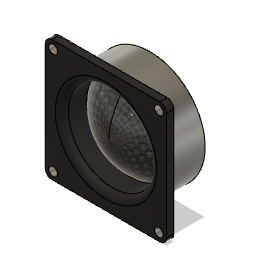
Main v23 (Autodesk Fusion 360 archive; units mm, degrees)
design "Monacor DT-28N"
Autodesk Fusion 360 part; units mm, degrees
sketch "Skizze1" plane through (0, 0, 0) normal (1, 0, 0) x (0, 0, -1)
  line L0 (16.7, 25) -> (16.7, 0)
  line L1 (16.7, 0) -> (0, 0)
  line L2 (16.7, 25) -> (-3.3, 25)
  line L3 (-3.3, 25) -> (-3.3, 23)
  line L4 (-0.3, 20) -> (8, 20)
  spline S0 degree 2 poles (8, 20) (-1.5, 11) (-2, 0) knots 0 0 0 2.280457 2.280457 2.280457
  arc A0 (-3.3, 23) -> (-0.3, 20) centre (-0.3, 23) ccw
  line L5 (0, 0) -> (-2, 0)
  dimension "d5" = 3.3
  dimension "d6" = 20
  dimension "d8" = 25
  dimension "d24" = 3
  dimension "d25" = 8
  dimension "d26" = 2
  dimension "d27" = 5
  dimension "d28" = 9
  dimension "d29" = 1.5
  constraint coincident L1.end L5.start
  constraint perpendicular L0 L1
  constraint perpendicular L0 L2
  constraint horizontal L2
  constraint perpendicular L2 L3
  constraint perpendicular L3 L4
  constraint tangent L3 A0
  constraint tangent L4 A0
  constraint parallel L1 L5
  measures "d5" horizontal distance of L1.end L2.end
  measures "d6" distance of L0.start L2.end
  measures "d8" vertical distance of L1.end L2.end
  measures "d24" radius of A0
  measures "d25" horizontal distance of L1.end L4.end
  measures "d26" distance of L1.end S0.end
  measures "d27" distance of L2 L4.end
revolve "Drehen1" add sketch "Skizze1" angle 360 about axis through (0, 0, 1.75) along (0, 0, 1)
sketch "Skizze2" plane through (0, 0, 3.3) normal (0, 0, 1) x (1, 0, 0)
  circle A0 centre (0, 0) radius 20
  circle A1 centre (0, 0) radius 25
  line L0 (24.5, -27.5) -> (-24.5, -27.5)
  line L1 (-27.5, -24.5) -> (-27.5, 24.5)
  line L2 (-24.5, 27.5) -> (24.5, 27.5)
  line L3 (27.5, 24.5) -> (27.5, -24.5)
  line L4 (27.5, -27.5) -> (-27.5, 27.5) construction
  line L5 (-27.5, -27.5) -> (27.5, 27.5) construction
  line L6 (24, -24) -> (-24, -24) construction
  line L7 (-24, -24) -> (-24, 24) construction
  line L8 (-24, 24) -> (24, 24) construction
  line L9 (24, 24) -> (24, -24) construction
  line L10 (24, -24) -> (-24, 24) construction
  line L11 (-24, -24) -> (24, 24) construction
  circle A2 centre (24, 24) radius 2
  circle A3 centre (-24, 24) radius 2
  circle A4 centre (-24, -24) radius 2
  circle A5 centre (24, -24) radius 2
  arc A6 (27.5, 24.5) -> (24.5, 27.5) centre (24.5, 24.5) ccw
  arc A7 (-24.5, 27.5) -> (-27.5, 24.5) centre (-24.5, 24.5) ccw
  arc A8 (-27.5, -24.5) -> (-24.5, -27.5) centre (-24.5, -24.5) ccw
  arc A9 (24.5, -27.5) -> (27.5, -24.5) centre (24.5, -24.5) ccw
  circle A10 centre (0, 0) radius 23
  circle A11 centre (0, 0) radius 25
  dimension "d11" = 55
  dimension "d12" = 55
  dimension "d13" = 48
  dimension "d14" = 48
  dimension "d15" = 4
  dimension "d17" = 360
  dimension "d18" = 3
  dimension "d19" = 3
  dimension "d20" = 3
  dimension "d21" = 3
  constraint perpendicular L0 L1
  constraint parallel L0 L2
  constraint parallel L1 L3
  constraint horizontal L0
  constraint coincident L4 A0.centre
  constraint coincident L5 A0.centre
  constraint coincident A0.centre A1.centre
  constraint perpendicular L6 L7
  constraint parallel L6 L8
  constraint parallel L7 L9
  constraint horizontal L6
  constraint coincident L10 A0.centre
  constraint coincident L11 A0.centre
  constraint coincident L8.end L9.start
  constraint coincident L5.end L3
  constraint coincident L5.end L2
  constraint tangent L3 A6
  constraint tangent L2 A6
  constraint coincident L4.end L2
  constraint coincident L4.end L1
  constraint tangent L2 A7
  constraint tangent L1 A7
  constraint coincident L5.start L1
  constraint coincident L5.start L0
  constraint tangent L1 A8
  constraint tangent L0 A8
  constraint coincident L4.start L0
  constraint coincident L4.start L3
  constraint tangent L0 A9
  constraint tangent L3 A9
  measures "d11" distance of L4.end L5.end
  measures "d12" distance of L5.start L4.end
  measures "d13" distance of L7.end L8.end
  measures "d14" distance of L6.end L7.end
  measures "d15" diameter of A2
  measures "d18" radius of A6
  measures "d19" radius of A7
  measures "d20" radius of A8
  measures "d21" radius of A9
extrude "Extrusion1" add sketch "Skizze2" against normal blind 3.3 contours L0 L1 L2 L3 A6 A7 A8 A9
named bodies: "Main"

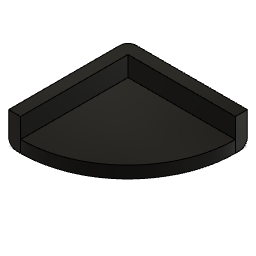
design "Corner"
Autodesk Fusion 360 part; units mm, degrees
sketch "Skizze1" plane through (0, 0, 0) normal (0, 1, 0) x (1, 0, 0)
  line L0 (0, 0) -> (0, -30)
  line L1 (0, 0) -> (30, 0)
  line L2 (0, -30) -> (3, -30)
  line L3 (3, -30) -> (3, -3)
  line L4 (3, -3) -> (30, -3)
  line L5 (30, -3) -> (30, 0)
  arc A0 (3, -30) -> (30, -3) centre (3, -3) ccw
  line L6 (3, -3) -> (3, -30) construction
  line L7 (3, -3) -> (30, -3) construction
  point P0 (3, -3)
  dimension "d1" = 30
  dimension "d2" = 30
  dimension "d4" = 27
  dimension "d5" = 27
  dimension "d6" = 90
  constraint coincident L0.start L1.start
  constraint vertical L0
  constraint horizontal L1
  constraint perpendicular L0 L2
  constraint perpendicular L2 L3
  constraint horizontal L4
  constraint vertical L5
  constraint coincident P0 L3.end
  measures "d1" distance of L0.start L0.end
  measures "d2" distance of L0.start L1.end
  measures "d4" distance of L2.end P0
  measures "d5" distance of P0 L4.end
  measures "d6" angle of L6 L7
extrude "Extrusion1" add sketch "Skizze1" against normal blind 3
extrude "Extrusion2" add sketch "Skizze1" along normal blind 5 contours L0 L1 L2 L3 L4 L5
fillet "Abrundung1" radius 2 3 edges at (0, 1, 0) (0, -3, 15) (15, -3, 0)
named bodies: "Main"

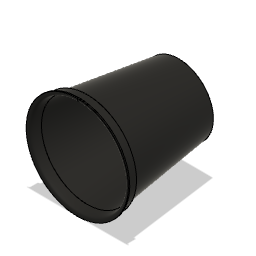
design "Monacor BR-100HP"
Autodesk Fusion 360 part; units mm, degrees
sketch "Skizze1" plane through (0, 0, 0) normal (1, 0, 0) x (0, 0, -1)
  line L0 (-1.8, 71.5) -> (0, 71.5)
  line L1 (0, 71.5) -> (0, 69)
  line L2 (0, 69) -> (12, 69)
  line L3 (12, 69) -> (12, 66)
  line L4 (12, 66) -> (140, 48.5186)
  line L5 (140, 48.5186) -> (140, 46.5)
  line L6 (140, 46.5) -> (12, 63.9814)
  spline S0 degree 2 poles (12, 63.9814) (-1.3, 65.7979) (-1.8, 71.5) knots 0 0 0 1.729263 1.729263 1.729263 weights 1 2.333333 1
  dimension "d1" = 71.5
  dimension "d2" = 2.5
  dimension "d3" = 3
  dimension "d4" = 2
  dimension "d5" = 140
  dimension "d6" = 1.8
  dimension "d7" = 12
  dimension "d8" = 46.5
  dimension "d9" = 1.3
  constraint perpendicular L0 L1
  constraint perpendicular L1 L2
  constraint perpendicular L2 L3
  constraint perpendicular L2 L5
  constraint parallel L4 L6
  constraint coincident origin L1
  constraint vertical L1
  constraint coincident L3 L6.end
  measures "d1" distance of origin L0.end
  measures "d2" distance of L0.end L1.end
  measures "d3" distance of L2.end L3.end
  measures "d4" distance of L4 L6
  measures "d5" horizontal distance of L0.end L4.end
  measures "d6" distance of L0.start L0.end
  measures "d7" distance of L1.end L2.end
  measures "d8" vertical distance of origin L5.end
revolve "Drehen1" add sketch "Skizze1" angle 360 about axis through (0, 0, 1.75) along (0, 0, 1)
equation "d1 = ( 143 / 2 ) * 1 mm"
equation "d2 = ( ( 143 - 138 ) / 2 ) * 1 mm"
equation "d8 = ( 93 / 2 ) * 1 mm"
named bodies: "Main"

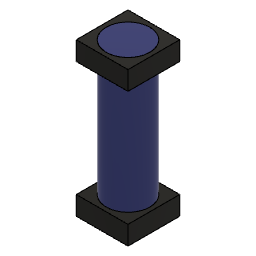
design "Cell"
Autodesk Fusion 360 part; units mm, degrees
sketch "Skizze1" plane through (0, 0, 0) normal (0, 1, 0) x (1, 0, 0)
  line L0 (11, -11) -> (-11, -11)
  line L1 (-11, -11) -> (-11, 11)
  line L2 (-11, 11) -> (11, 11)
  line L3 (11, 11) -> (11, -11)
  line L4 (11, -11) -> (-11, 11) construction
  line L5 (-11, -11) -> (11, 11) construction
  circle A0 centre (0, 0) radius 9.25
  dimension "d1" = 22
  dimension "d2" = 22
  dimension "d3" = 18.5
  constraint perpendicular L0 L1
  constraint parallel L0 L2
  constraint parallel L1 L3
  constraint horizontal L0
  constraint coincident L4 A0.centre
  constraint coincident L5 A0.centre
  constraint coincident A0.centre origin
  measures "d1" distance of L0.end L1.end
  measures "d2" distance of L1.end L2.end
  measures "d3" diameter of A0
extrude "Extrusion1" add sketch "Skizze1" along normal blind 65 contours A0 makes body 1
extrude "Extrusion2" add sketch "Skizze1" along normal blind 8 separate body makes body 2
copy_body "Körper kopieren/einfügen1" bodies 2 makes body 3
move_body "Verschieben2" bodies 3 to x (1, 0, 0) y (0, 1, 0) z (0, 0, 1) at (0, 57, 0)

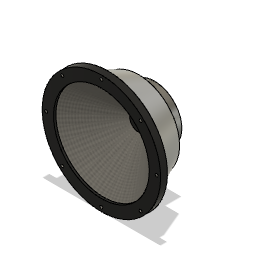
design "Beyma 10BR60V2"
Autodesk Fusion 360 part; units mm, degrees
sketch "Skizze1" plane through (0, 0, 0) normal (1, 0, 0) x (0, 0, -1)
  line L0 (67, 20) -> (67, 0)
  line L1 (67, 0) -> (102, 0)
  line L2 (102, 0) -> (102, 60)
  line L3 (102, 60) -> (67, 60)
  line L4 (-15, 130.25) -> (-15, 105.25)
  line L5 (-15, 105.25) -> (-10, 105.25)
  line L6 (-10, 105.25) -> (67, 20)
  line L7 (0, 130.25) -> (0, 114)
  line L8 (0, 130.25) -> (-15, 130.25)
  line L9 (67, 60) -> (67, 90)
  line L10 (0, 114) -> (10, 114)
  line L11 (10, 114) -> (67, 90)
  dimension "d1" = 114
  dimension "d2" = 20
  dimension "d4" = 15
  dimension "d5" = 5
  dimension "d7" = 16.25
  dimension "d8" = 102
  dimension "d9" = 35
  dimension "d10" = 60
  dimension "d11" = 30
  dimension "d12" = 25
  dimension "d22" = 10
  constraint perpendicular L0 L1
  constraint perpendicular L1 L2
  constraint perpendicular L2 L3
  constraint perpendicular L4 L5
  constraint coincident origin L1
  constraint perpendicular L4 L8
  constraint vertical L7
  constraint horizontal L8
  constraint coincident origin L7
  constraint horizontal L3
  constraint perpendicular L3 L9
  constraint collinear L0 L9
  constraint perpendicular L7 L10
  measures "d1" vertical distance of origin L7.end
  measures "d2" vertical distance of origin L0.start
  measures "d4" distance of L7.start L4.start
  measures "d5" distance of L4.end L5.end
  measures "d7" distance of L7.start L7.end
  measures "d8" distance of origin L1.end
  measures "d9" distance of L2.end L3.end
  measures "d10" distance of L1.end L2.end
  measures "d11" distance of L3.end L9.end
  measures "d12" distance of L4.start L4.end
  measures "d22" distance of L7.end L10.end
revolve "Drehen1" add sketch "Skizze1" angle 360 about axis through (0, 0, 1.75) along (0, 0, 1)
sketch "Skizze2" plane through (0, 0, 15) normal (0, 0, 1) x (1, 0, 0)
  circle A0 centre (0, 0) radius 105.25
  circle A1 centre (0, 0) radius 130.25
  circle A2 centre (0, 0) radius 121.75 construction
  circle A3 centre (0, 121.75) radius 3.1
  line L0 (0, 0) -> (0, 140) construction
  circle A4 centre (-86.0903, 86.0903) radius 3.1
  circle A5 centre (-121.75, 0) radius 3.1
  circle A6 centre (-86.0903, -86.0903) radius 3.1
  circle A7 centre (0, -121.75) radius 3.1
  circle A8 centre (86.0903, -86.0903) radius 3.1
  circle A9 centre (121.75, 0) radius 3.1
  circle A10 centre (86.0903, 86.0903) radius 3.1
  dimension "d14" = 243.5
  dimension "d16" = 6.2
  dimension "d17" = 140
  dimension "d19" = 360
  constraint coincident A0.centre A1.centre
  constraint coincident A2 A3.centre
  constraint vertical L0
  constraint coincident A3.centre L0
  measures "d14" diameter of A2
  measures "d16" diameter of A3
  measures "d17" distance of A0.centre L0.end
extrude "Extrusion1" cut sketch "Skizze2" against normal blind 20 contours A3 | A4 | A5 | A6 | A7 | A8 | A9 | A10
equation "d1 = ( 228 / 2 ) * 1 mm"
named bodies: "Main"

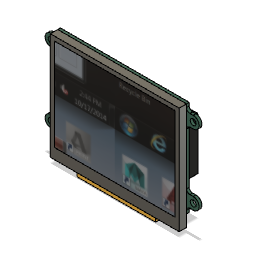
design "NHD-3.5-320240FT-CSXN-T"
Autodesk Fusion 360 part; units mm, degrees
sketch "Skizze1" plane through (0, 0, 0) normal (0, 0, 1) x (1, 0, 0)
  line L0 (0, 0) -> (76.9, 0)
  line L1 (76.9, 0) -> (76.9, 63.9)
  line L2 (76.9, 63.9) -> (0, 63.9)
  line L3 (0, 63.9) -> (0, 0)
  line L4 (0, 31.95) -> (76.9, 31.95) construction
  line L5 (0, 35.45) -> (76.9, 35.45) construction
  circle A0 centre (-4, 14.45) radius 1.75
  line L6 (38.45, 0) -> (38.45, 63.9) construction
  line L7 (74.36, 6.31) -> (2.54, 6.31)
  line L8 (2.54, 6.31) -> (2.54, 61.36)
  line L9 (2.54, 61.36) -> (74.36, 61.36)
  line L10 (74.36, 61.36) -> (74.36, 6.31)
  line L11 (74.36, 6.31) -> (2.54, 61.36) construction
  line L12 (2.54, 6.31) -> (74.36, 61.36) construction
  line L13 (15, 0) -> (15, -3)
  line L14 (15, -3) -> (61.9, -3)
  line L15 (61.9, -3) -> (61.9, 0)
  line L16 (76.9, 7) -> (0, 7)
  line L17 (15, 7) -> (15, 0)
  line L18 (61.9, 0) -> (61.9, 7)
  line L19 (-2, 18) -> (-4, 18)
  arc A1 (-4, 18) -> (-7.55, 14.45) centre (-4, 14.45) ccw
  line L20 (-4, 14.45) -> (-4, 18) construction
  line L21 (-4, 14.45) -> (-7.55, 14.45) construction
  arc A2 (-7.55, 14.45) -> (-4, 10.9) centre (-4, 14.45) ccw
  line L22 (-4, 14.45) -> (-7.55, 14.45) construction
  line L23 (-4, 14.45) -> (-4, 10.9) construction
  line L24 (-4, 10.9) -> (-2, 10.9)
  arc A3 (-2, 18) -> (0, 20) centre (-2, 20) ccw
  arc A4 (0, 8.9) -> (-2, 10.9) centre (-2, 8.9) ccw
  arc A5 (-4, 60) -> (-7.55, 56.45) centre (-4, 56.45) ccw
  line L25 (-4, 56.45) -> (-7.55, 56.45) construction
  arc A6 (-2, 60) -> (0, 62) centre (-2, 62) ccw
  line L26 (-4, 56.45) -> (-4, 52.9) construction
  arc A7 (0, 50.9) -> (-2, 52.9) centre (-2, 50.9) ccw
  circle A8 centre (-4, 56.45) radius 1.75
  line L27 (-4, 56.45) -> (-4, 60) construction
  line L28 (-4, 56.45) -> (-7.55, 56.45) construction
  line L29 (-2, 52.9) -> (-4, 52.9)
  line L30 (-4, 60) -> (-2, 60)
  arc A9 (-7.55, 56.45) -> (-4, 52.9) centre (-4, 56.45) ccw
  line L31 (80.9, 14.45) -> (84.45, 14.45) construction
  line L32 (78.9, 18) -> (80.9, 18)
  circle A10 centre (80.9, 14.45) radius 1.75
  arc A11 (84.45, 14.45) -> (80.9, 18) centre (80.9, 14.45) ccw
  line L33 (80.9, 14.45) -> (84.45, 14.45) construction
  arc A12 (78.9, 10.9) -> (76.9, 8.9) centre (78.9, 8.9) ccw
  line L34 (80.9, 14.45) -> (80.9, 10.9) construction
  line L35 (80.9, 14.45) -> (80.9, 18) construction
  arc A13 (76.9, 20) -> (78.9, 18) centre (78.9, 20) ccw
  line L36 (80.9, 10.9) -> (78.9, 10.9)
  arc A14 (80.9, 10.9) -> (84.45, 14.45) centre (80.9, 14.45) ccw
  line L37 (80.9, 56.45) -> (84.45, 56.45) construction
  arc A15 (78.9, 52.9) -> (76.9, 50.9) centre (78.9, 50.9) ccw
  line L38 (80.9, 56.45) -> (84.45, 56.45) construction
  arc A16 (84.45, 56.45) -> (80.9, 60) centre (80.9, 56.45) ccw
  arc A17 (80.9, 52.9) -> (84.45, 56.45) centre (80.9, 56.45) ccw
  line L39 (80.9, 56.45) -> (80.9, 52.9) construction
  line L40 (80.9, 60) -> (78.9, 60)
  arc A18 (76.9, 62) -> (78.9, 60) centre (78.9, 62) ccw
  line L41 (78.9, 52.9) -> (80.9, 52.9)
  line L42 (80.9, 56.45) -> (80.9, 60) construction
  circle A19 centre (80.9, 56.45) radius 1.75
  point P0 (-2, 62)
  point P1 (76.9, 31.95)
  point P2 (76.9, 35.45)
  point P3 (38.45, 33.835)
  point P4 (78.9, 62)
  dimension "d1" = 76.9
  dimension "d2" = 63.9
  dimension "d18" = 28.45
  dimension "d23" = 3.5
  dimension "d24" = 21
  dimension "d26" = 42.45
  dimension "d29" = 71.82
  dimension "d30" = 55.05
  dimension "d31" = 2.54
  dimension "d34" = 3
  dimension "d35" = 15
  dimension "d36" = 7
  dimension "d39" = 46
  dimension "d40" = 15.45
  constraint horizontal L0
  constraint horizontal L2
  constraint vertical L3
  constraint coincident L0.start L3.end
  constraint midpoint L3 L4.start
  constraint midpoint L1 P1
  constraint coincident L3 L5.start
  constraint coincident L1 P2
  constraint perpendicular L1 L5
  constraint midpoint L0 L6.start
  constraint midpoint L2 L6.end
  constraint symmetric L4.start L6 P1
  constraint symmetric L5.start L6 P2
  constraint perpendicular L7 L8
  constraint parallel L7 L9
  constraint parallel L8 L10
  constraint horizontal L7
  constraint coincident L11 P3
  constraint coincident L12 P3
  constraint coincident L6 P3
  constraint coincident L0 L13.start
  constraint perpendicular L0 L13
  constraint perpendicular L13 L14
  constraint coincident L0 L15.end
  constraint perpendicular L0 L15
  constraint symmetric L6 L13 L15
  constraint coincident L1 L16.start
  constraint coincident L3 L16.end
  constraint perpendicular L3 L16
  constraint coincident L16 L18.end
  constraint perpendicular L16 L18
  constraint coincident L16 L17.start
  constraint collinear L13 L17
  constraint coincident A0.centre A1.centre
  constraint vertical L20
  constraint horizontal L21
  constraint vertical L23
  constraint tangent L19 A1
  constraint tangent A2 L24
  constraint coincident L3 A3.end
  constraint tangent L19 A3
  constraint tangent L3 A3
  constraint coincident L3 A4.start
  constraint tangent L24 A4
  constraint tangent L3 A4
  constraint equal L19 L24
  constraint symmetric L5 L19.start A7.end
  constraint symmetric L5 A0 A8
  constraint symmetric L5 L24.end A6.start
  constraint symmetric L5 L19.end L26.end
  constraint symmetric L5 A1.end A5.end
  constraint symmetric L5 A1 A9
  constraint symmetric L5 A2.end A5.start
  constraint symmetric L5 A2 A5
  constraint symmetric L5 A3.end A7.start
  constraint symmetric L5 A3 A7
  constraint symmetric L5 A4.start A6.end
  constraint symmetric L5 A4 A6
  constraint symmetric L19.start L6 L32.start
  constraint symmetric A0 L6 A10
  constraint symmetric L6 L24.end A12.start
  constraint symmetric L6 P0 P4
  constraint symmetric L6 L19.end L32.end
  constraint symmetric L6 A1.end L31.end
  constraint symmetric L6 A1 A11
  constraint symmetric L6 A2.end L34.end
  constraint symmetric L6 A2 A14
  constraint symmetric L6 A3.end A13.start
  constraint symmetric L6 A3 A13
  constraint symmetric L6 A4.start A12.end
  constraint symmetric L6 A4 A12
  constraint symmetric L6 A5.end L37.end
  constraint symmetric L6 L26.end A17.start
  constraint symmetric L6 A6.start L40.end
  constraint symmetric L6 A7.start A15.end
  constraint symmetric L6 A7.end A15.start
  constraint symmetric L6 A6.end A18.start
  constraint symmetric L6 A5.start A16.end
  constraint symmetric L6 A5 A16
  constraint symmetric L6 A6 A18
  constraint symmetric L6 A7 A15
  constraint symmetric L6 A8 A19
  constraint symmetric L6 A9 A17
  measures "d1" distance of L0.start L0.end
  measures "d2" distance of L0.start L2.end
  measures "d18" distance of L2 L5
  measures "d23" diameter of A0
  measures "d24" distance of L5 A0.centre
  measures "d26" distance of A0.centre L6
  measures "d29" distance of L8.end L9.end
  measures "d30" distance of L7.end L8.end
  measures "d31" distance of L2 L8.end
  measures "d34" distance of L13.start L13.end
  measures "d35" distance of L0.start L13.start
  measures "d36" distance of L0.start L16.end
  measures "d39" distance of L6 A1.end
  measures "d40" distance of L5 A3.end
extrude "Extrusion3" add sketch "Skizze1" along normal blind 3.5 contours L0 L13 L14 L15 makes body 1
extrude "Extrusion4" add sketch "Skizze1" against normal blind 1.6 contours L0 L7 L17 L18 | L0 L13 L14 L15 | L7 L16 L17 L18 bodies 1
extrude "Extrusion5" add sketch "Skizze1" against normal blind 1.6 separate body contours L1 L2 L3 L8 L9 L10 L16 | L3 L19 A1 A2 L24 A3 A4 | L8 L9 L10 L16 | L3 A5 A6 A7 L29 L30 A9 | L1 L32 A11 A12 A13 L36 A14 | L1 A15 A16 A17 L40 A18 L41 makes body 2
extrude "Extrusion6" add sketch "Skizze1" along normal blind 4.4 separate body contours L0 L3 L7 L8 L16 L17 | L0 L7 L17 L18 | L1 L2 L3 L8 L9 L10 L16 | L0 L1 L7 L10 L16 L18 makes body 3
extrude "Extrusion7" add sketch "Skizze1" along normal blind 4.4 separate body contours L7 L16 L17 L18 | L7 L8 L16 L17 | L8 L9 L10 L16 | L7 L10 L16 L18 makes body 4
sketch "Skizze2" plane through (0, 0, -1.6) normal (0, 0, -1) x (-1, 0, 0)
  circle A0 centre (4, 14.45) radius 1.75
  circle A1 centre (-80.9, 56.45) radius 1.75
  circle A2 centre (4, 56.45) radius 1.75
  circle A3 centre (-80.9, 14.45) radius 1.75
  line L0 (-76.9, 50.9) -> (-76.9, 20)
  arc A4 (-78.9, 18) -> (-76.9, 20) centre (-78.9, 20) ccw
  line L1 (-78.9, 18) -> (-80.9, 18)
  arc A5 (-80.9, 18) -> (-80.9, 10.9) centre (-80.9, 14.45) ccw
  line L2 (-80.9, 10.9) -> (-78.9, 10.9)
  arc A6 (-76.9, 8.9) -> (-78.9, 10.9) centre (-78.9, 8.9) ccw
  line L3 (-76.9, 8.9) -> (-76.9, 7)
  line L4 (-76.9, 7) -> (0, 7)
  line L5 (0, 7) -> (0, 8.9)
  arc A7 (2, 10.9) -> (0, 8.9) centre (2, 8.9) ccw
  line L6 (2, 10.9) -> (4, 10.9)
  arc A8 (4, 10.9) -> (4, 18) centre (4, 14.45) ccw
  line L7 (4, 18) -> (2, 18)
  arc A9 (0, 20) -> (2, 18) centre (2, 20) ccw
  line L8 (0, 20) -> (0, 50.9)
  arc A10 (2, 52.9) -> (0, 50.9) centre (2, 50.9) ccw
  line L9 (2, 52.9) -> (4, 52.9)
  arc A11 (4, 52.9) -> (4, 60) centre (4, 56.45) ccw
  line L10 (4, 60) -> (2, 60)
  arc A12 (0, 62) -> (2, 60) centre (2, 62) ccw
  line L11 (0, 62) -> (0, 63.9)
  line L12 (0, 63.9) -> (-76.9, 63.9)
  line L13 (-76.9, 63.9) -> (-76.9, 62)
  arc A13 (-78.9, 60) -> (-76.9, 62) centre (-78.9, 62) ccw
  line L14 (-78.9, 60) -> (-80.9, 60)
  arc A14 (-80.9, 60) -> (-80.9, 52.9) centre (-80.9, 56.45) ccw
  line L15 (-80.9, 52.9) -> (-78.9, 52.9)
  arc A15 (-76.9, 50.9) -> (-78.9, 52.9) centre (-78.9, 50.9) ccw
  line L16 (-72.4, 50.9) -> (-64.4, 50.9)
  line L17 (-64.4, 50.9) -> (-64.4, 20)
  line L18 (-64.4, 20) -> (-72.4, 20)
  line L19 (-72.4, 20) -> (-72.4, 50.9)
  line L20 (-76.9, 35.45) -> (0, 35.45) construction
  line L21 (-61.9, 50.9) -> (-15, 50.9)
  line L22 (-15, 50.9) -> (-15, -3)
  line L23 (-15, -3) -> (-61.9, -3)
  line L24 (-61.9, -3) -> (-61.9, 50.9)
  line L25 (0, 47.95) -> (-7, 47.95)
  line L26 (-7, 47.95) -> (-7, 22.95)
  line L27 (-7, 22.95) -> (0, 22.95)
  line L28 (0, 22.95) -> (0, 47.95)
  point P0 (-72.4, 35.45)
  point P1 (-61.9, -3)
  point P2 (-15, -3)
  dimension "d55" = 8
  dimension "d56" = 30.9
  dimension "d57" = 4.5
  dimension "d58" = 7
  dimension "d59" = 25
  constraint horizontal L16
  constraint vertical L17
  constraint horizontal L18
  constraint vertical L19
  constraint midpoint L0 L20.start
  constraint midpoint L8 L20.end
  constraint midpoint L19 P0
  constraint coincident L20 P0
  constraint horizontal L21
  constraint vertical L22
  constraint horizontal L23
  constraint vertical L24
  constraint coincident P1 L23.end
  constraint coincident P2 L22.end
  constraint collinear L16 L21
  constraint horizontal L25
  constraint vertical L26
  constraint horizontal L27
  constraint vertical L28
  constraint coincident L8 L25.start
  constraint midpoint L20.end L28
  measures "d55" distance of L16.start L16.end
  measures "d56" distance of L16.start L18.end
  measures "d57" distance of L0 L18.end
  measures "d58" distance of L26.end L27.end
  measures "d59" distance of L25.end L26.end
extrude "Extrusion8" add sketch "Skizze2" along normal blind 9.8 separate body contours L16 L17 L18 L19 makes body 5
extrude "Extrusion9" add sketch "Skizze2" along normal blind 2 separate body contours L8 L25 L26 L27 L28 makes body 6
extrude "Extrusion10" add sketch "Skizze2" along normal blind 2 separate body contours L4 L21 L22 L24 | L4 L22 L23 L24 makes body 7
combine "Kombinieren1" operation add target body 1 tool bodies 7
equation "d26 = ( 84.9 / 2 ) * 1 mm"
equation "d36 = 63.9 mm - 56.9 mm"
equation "d39 = ( 92 / 2 ) * 1 mm"
equation "d40 = ( 30.9 / 2 ) * 1 mm"
equation "d60 = 11.4 mm - 1.6 mm"
named bodies: "FFCPlaceholder", "PCB", "MetalFrame", "LCD", "IDC Connector", "FFC Connector"

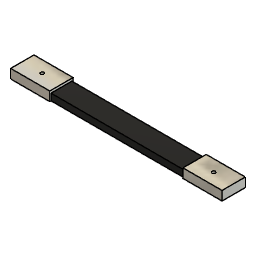
design "Handle"
Autodesk Fusion 360 part; units mm, degrees
sketch "Skizze1" plane through (0, 0, 0) normal (0, 1, 0) x (1, 0, 0)
  line L0 (80, -12.5) -> (-80, -12.5)
  line L1 (-80, -12.5) -> (-80, 12.5)
  line L2 (-80, 12.5) -> (80, 12.5)
  line L3 (80, 12.5) -> (80, -12.5)
  line L4 (80, -12.5) -> (-80, 12.5) construction
  line L5 (-80, -12.5) -> (80, 12.5) construction
  line L6 (80, 14) -> (127, 14)
  line L7 (127, 14) -> (127, -14)
  line L8 (127, -14) -> (80, -14)
  line L9 (80, -14) -> (80, 14)
  line L10 (0, 12.5) -> (0, -12.5) construction
  line L11 (80, 0) -> (127, 0) construction
  circle A0 centre (103, 0) radius 2
  line L12 (-80, 0) -> (-127, 0) construction
  line L13 (-127, -14) -> (-80, -14)
  circle A1 centre (-103, 0) radius 2
  line L14 (-127, 14) -> (-127, -14)
  line L15 (-80, 14) -> (-127, 14)
  line L16 (-80, -14) -> (-80, 14)
  dimension "d1" = 160
  dimension "d2" = 25
  dimension "d3" = 28
  dimension "d4" = 47
  dimension "d5" = 4
  dimension "d6" = 103
  constraint perpendicular L0 L1
  constraint parallel L0 L2
  constraint parallel L1 L3
  constraint horizontal L0
  constraint coincident L4 origin
  constraint coincident L5 origin
  constraint horizontal L6
  constraint vertical L7
  constraint horizontal L8
  constraint vertical L9
  constraint midpoint L3 L9
  constraint midpoint L2 L10.start
  constraint midpoint L0 L10.end
  constraint midpoint L9 L11.start
  constraint midpoint L7 L11.end
  constraint coincident L11 A0.centre
  constraint symmetric L6.start L10 L15.start
  constraint symmetric L6.end L10 L14.start
  constraint symmetric L7.end L10 L13.start
  constraint symmetric L8.end L10 L13.end
  constraint symmetric L10 L11.start L12.start
  constraint symmetric L10 L11.end L12.end
  constraint symmetric L10 A0 A1
  measures "d1" distance of L1.end L2.end
  measures "d2" distance of L0.end L1.end
  measures "d3" distance of L6.start L8.end
  measures "d4" distance of L6.start L6.end
  measures "d5" diameter of A0
  measures "d6" distance of origin A0.centre
extrude "Extrusion1" add sketch "Skizze1" along normal blind 11 contours L3 L6 L7 L8 L9 | L1 L13 L14 L15 L16 makes body 1 at (-119.6667, 0, 0) makes body 2 at (119.6667, 0, 0)
extrude "Extrusion2" add sketch "Skizze1" along normal blind 8 separate body contours L0 L1 L2 L3 L9 L16 makes body 3
equation "d4 = ( ( 254 - 160 ) / 2 ) * 1 mm"
named bodies: "End1", "End2", "Center"

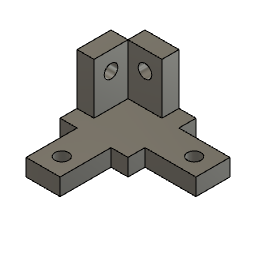
design "2020 Corner Piece"
Autodesk Fusion 360 part; units mm, degrees
sketch "Skizze1" plane through (0, 0, 0) normal (0, 1, 0) x (1, 0, 0)
  line L0 (0, 0) -> (20, 0)
  line L1 (0, 0) -> (0, -20)
  line L2 (0, -20) -> (5, -20)
  line L3 (5, -20) -> (5, -35)
  line L4 (5, -35) -> (15, -35)
  line L5 (15, -35) -> (15, -20)
  line L6 (15, -20) -> (20, -20)
  line L7 (20, -20) -> (20, -15)
  line L8 (20, -15) -> (35, -15)
  line L9 (35, -15) -> (35, -5)
  line L10 (35, -5) -> (20, -5)
  line L11 (20, -5) -> (20, 0)
  line L12 (35, -10) -> (0, -10) construction
  line L13 (10, 0) -> (10, -35) construction
  circle A0 centre (29.5, -10) radius 2
  circle A1 centre (10, -29.5) radius 2
  dimension "d3" = 20
  dimension "d4" = 20
  dimension "d5" = 5
  dimension "d6" = 15
  dimension "d7" = 10
  dimension "d8" = 15
  dimension "d9" = 10
  dimension "d10" = 5
  dimension "d11" = 4
  dimension "d12" = 5.5
  dimension "d13" = 4
  dimension "d14" = 5.5
  constraint horizontal L0
  constraint coincident L0.start L1.start
  constraint perpendicular L0 L1
  constraint perpendicular L1 L2
  constraint perpendicular L2 L3
  constraint perpendicular L3 L4
  constraint perpendicular L4 L5
  constraint perpendicular L5 L6
  constraint perpendicular L6 L7
  constraint perpendicular L7 L8
  constraint perpendicular L8 L9
  constraint perpendicular L9 L10
  constraint collinear L2 L6
  constraint collinear L7 L11
  constraint midpoint L9 L12.start
  constraint midpoint L1 L12.end
  constraint midpoint L0 L13.start
  constraint midpoint L4 L13.end
  constraint coincident L12 A0.centre
  constraint coincident L13 A1.centre
  measures "d3" distance of L0.start L0.end
  measures "d4" distance of L0.start L1.end
  measures "d5" distance of L1.end L2.end
  measures "d6" distance of L2.end L3.end
  measures "d7" distance of L3.end L4.end
  measures "d8" distance of L7.end L8.end
  measures "d9" distance of L8.end L9.end
  measures "d10" distance of L0.end L10.end
  measures "d11" diameter of A0
  measures "d12" distance of L9 A0.centre
  measures "d13" diameter of A1
  measures "d14" distance of L4 A1.centre
extrude "Extrusion1" add sketch "Skizze1" along normal blind 5
sketch "Skizze3" plane through (0, 0, 0) normal (0, 0, -1) x (-1, 0, 0)
  line L0 (-20, 0) -> (0, 0)
  line L1 (0, 0) -> (0, 5)
  line L2 (0, 5) -> (-20, 5)
  line L3 (-20, 5) -> (-20, 0)
  line L4 (-5, 5) -> (-15, 5)
  line L5 (-15, 5) -> (-15, 20)
  line L6 (-15, 20) -> (-5, 20)
  line L7 (-5, 20) -> (-5, 5)
  line L8 (-10, 5) -> (-10, 20) construction
  circle A0 centre (-10, 14.5) radius 2
  dimension "d17" = 10
  dimension "d18" = 15
  dimension "d19" = 5
  dimension "d20" = 4
  dimension "d21" = 5.5
  constraint horizontal L4
  constraint vertical L5
  constraint horizontal L6
  constraint vertical L7
  constraint coincident L2 L4.start
  constraint midpoint L4 L8.start
  constraint midpoint L6 L8.end
  constraint coincident L8 A0.centre
  measures "d17" distance of L4.start L4.end
  measures "d18" distance of L4.start L6.end
  measures "d19" horizontal distance of L0.end L4.start
  measures "d20" diameter of A0
  measures "d21" distance of L6 A0.centre
sketch "Skizze4" plane through (0, 0, 0) normal (-1, 0, 0) x (0, 0, 1)
  line L0 (0, 0) -> (20, 0)
  line L1 (20, 0) -> (20, 5)
  line L2 (20, 5) -> (0, 5)
  line L3 (0, 5) -> (0, 0)
  line L4 (5, 5) -> (15, 5)
  line L5 (15, 5) -> (15, 20)
  line L6 (15, 20) -> (5, 20)
  line L7 (5, 20) -> (5, 5)
  line L8 (10, 20) -> (10, 5) construction
  circle A0 centre (10, 14.5) radius 2
  dimension "d22" = 10
  dimension "d23" = 15
  dimension "d24" = 5
  dimension "d25" = 4
  dimension "d26" = 5.5
  constraint horizontal L4
  constraint vertical L5
  constraint horizontal L6
  constraint vertical L7
  constraint coincident L2 L4.start
  constraint midpoint L6 L8.start
  constraint midpoint L4 L8.end
  constraint coincident L8 A0.centre
  measures "d22" distance of L4.start L4.end
  measures "d23" distance of L4.start L6.end
  measures "d24" horizontal distance of L4.start L0.start
  measures "d25" diameter of A0
  measures "d26" distance of L6 A0.centre
extrude "Extrusion2" add sketch "Skizze3" against normal blind 5 contours L2 L4 L5 L6 L7
extrude "Extrusion4" add sketch "Skizze4" against normal blind 5 contours L2 L4 L5 L6 L7
named bodies: "Main"
